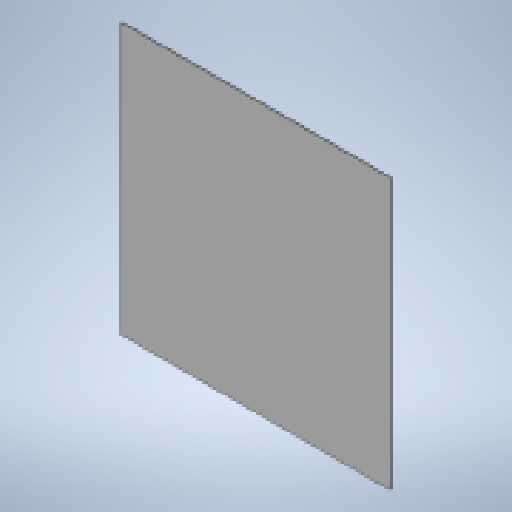
# Autodesk Inventor part: CH 1019 GBK shield
Saved by Autodesk Inventor 2026 (Build 300175000, 175)
## iProperties
Created: 2026-04-17
Part Number: CH 1019 GBK shield
Material: Steel
Document SubType Name: Sheet Metal
Designer: pokla
Density: 7.85 g/cm^3
Sheet Metal Rule: По умолчанию_мм
Appearance: Default
Mass: 69243.3 g
Surface Area: 44341.6 cm^2
Volume: 8820.8 cm^3
Flat Pattern Width: 148 cm
Flat Pattern Length: 149 cm
Flat Pattern Area: 22052 cm^2
Sheet Metal Width: 1480,000 мм
Sheet Metal Length: 1490,000 мм
Sheet Metal Area: 2205200,000 мм^2
Stock Number: 1318
Author: admin
Autodesk Inventor part; units mm, degrees
ref_plane "YZ Plane" through (0, 0, 0) normal (1, 0, 0) x (0, 1, 0)
ref_plane "XZ Plane" through (0, 0, 0) normal (0, 1, 0) x (-1, 0, 0)
ref_plane "XY Plane" through (0, 0, 0) normal (0, 0, 1) x (1, 0, 0)
sketch "Sketch1" plane through (0, 0, 0) normal (0, 0, 1) x (1, 0, 0)
  line L0 (740, -745) -> (-740, -745)
  line L1 (-740, -745) -> (-740, 745)
  line L2 (-740, 745) -> (740, 745)
  line L3 (740, 745) -> (740, -745)
  line L4 (740, -745) -> (-740, 745) construction
  line L5 (-740, -745) -> (740, 745) construction
  point P0 (0, 0)
  dimension "d0" = 1480
  dimension "d1" = 1490
  measures "d0" distance of L1.end L2.end
  measures "d1" distance of L0.end L1.end
extrude "Plate1" add sketch "Sketch1" along normal blind 4
sketch "Sketch2" plane through (0, 0, 0) normal (0, 0, -1) x (-1, 0, 0)
  line L0 (525.2603, -544.1907) -> (525.2603, -1005.879) construction
  line L1 (525.2603, -1005.879) -> (495.2603, -1005.879) construction
  line L2 (495.2603, -1005.879) -> (495.2603, -544.1907) construction
  line L3 (495.2603, -544.1907) -> (525.2603, -544.1907) construction
  line L4 (710, -491) -> (710, -487) projected
  line L5 (710, 5.6667) -> (710, 9.6667) projected
  line L6 (710, 502.3333) -> (710, 506.3333) projected
  line L7 (230.5109, -494.5) -> (230.5109, -591.5) projected
  line L8 (230.5109, -591.5) -> (226.5119, -591.5) projected
  line L9 (-269.6177, -494.5) -> (-269.6177, -591.5) projected
  line L10 (-269.6177, -591.5) -> (-273.6167, -591.5) projected
  line L11 (-739.3197, -491) -> (-710, -491) projected
  line L12 (-710, -491) -> (-710, -487) projected
  line L13 (-739.3197, 5.6667) -> (-710, 5.6667) projected
  line L14 (-710, 5.6667) -> (-710, 9.6667) projected
  line L15 (-739.3197, 502.3333) -> (-710, 502.3333) projected
  line L16 (-710, 502.3333) -> (-710, 506.3333) projected
  ellipse E0 centre (-269.6177, 743.5) end of major axis (-269.6177, 773.5) minor radius 0.6803 (-269.6177, 713.5) -> (-269.6177, 773.5) ccw projected
  line L17 (-269.6177, 713.5) -> (-273.6167, 713.5) projected
  ellipse E1 centre (230.5109, 743.5) end of major axis (230.5109, 773.5) minor radius 0.6803 (230.5109, 713.5) -> (230.5109, 773.5) ccw projected
  line L18 (230.5109, 713.5) -> (226.5119, 713.5) projected
  line L19 (710, -491) -> (680, -491)
  line L20 (710, 5.6667) -> (680, 5.6667)
  line L21 (710, 502.3333) -> (680, 502.3333)
  point P0 (0, 0)
  dimension "d3" = 30
  dimension "d4" = 30
  dimension "d5" = 30
  constraints: 6 end point, 3 horizontal, 4 other
  measures "d3" distance of L4.start L19.end
  measures "d4" distance of L20.start L20.end
  measures "d5" distance of L21.start L21.end
mark "Mark1"
equation "\"d0\" = Лист_ширина"
equation "\"d2\" = Thickness"
equation "\"BendRadius\" = Thickness"
equation "\"BendReliefWidth\" = Thickness"
equation "\"BendReliefDepth\" = 0.5 * Thickness"
equation "\"CornerReliefSize\" = 4 * Thickness"
equation "\"MinimumRemnant\" = 2 * Thickness"
equation "\"TransitionRadius\" = BendRadius"
equation "\"JacobiRadiusSize\" = BendRadius"
equation "\"GapSize\" = Thickness"
equation "\"Лист_ширина\" = 1480"
equation "\"Thickness\" = 4"
body "Solid1"
